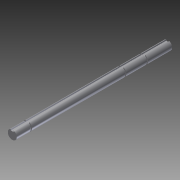
# Autodesk Inventor part: vertical drive shaft
Saved by Autodesk Inventor 2012 (Build 160160000, 160)
## iProperties
Created: 2012-07-07
Part Number: vertical drive shaft
Material: Default
Document SubType Name: Modeling
Designer: Bryce
Density: 1 g/cm^3
Author: Bryce
Autodesk Inventor part; units mm, degrees
sketch "Sketch1" plane through (0, 0, 0) normal (0, 0, 1) x (1, 0, 0)
  circle A0 centre (0, 0) radius 4.7625
  line L0 (-1.5875, 6.35) -> (1.5875, 6.35)
  line L1 (1.5875, 6.35) -> (1.5875, 3.175)
  line L2 (1.5875, 3.175) -> (-1.5875, 3.175)
  line L3 (-1.5875, 3.175) -> (-1.5875, 6.35)
  dimension "d0" = 9.525
  dimension "d43" = 3.175
  dimension "d44" = 3.175
  dimension "d45" = 1.5875
  dimension "d46" = 6.35
  constraints: 8 end point, 2 parallel, 1 centre point, 1 coincident, 1 horizontal, 1 perpendicular
  measures "d0" diameter of A0
  measures "d43" distance of L0.start L0.end
  measures "d44" distance of L0.end L1.end
  measures "d45" distance from line of point (0, 0) L1
  measures "d46" distance from line of point (0, 0) L0
extrude "Extrusion1" add sketch "Sketch1" along normal blind 165.05 contours A0 L3 L2 L1 | L1 L2 L3 A0
ref_plane "Work Plane6" through (0, 0, 176.4284) normal (0, 0, 1) x (1, 0, 0)
ref_plane "Work Plane12" through (0, 0, 148.9464) normal (0, 0, 1) x (1, 0, 0)
sketch "Sketch10" plane through (0, 0, 148.9464) normal (0, 0, 1) x (1, 0, 0)
  circle A0 centre (0, 0) radius 3.8481 projected
  circle A1 centre (0, 0) radius 4.7625 projected
extrude "Extrusion11" cut sketch "Sketch10" along normal blind 1.143
ref_plane "Work Plane13" through (0, 0, 49.7586) normal (0, 0, -1) x (-1, 0, 0)
sketch "Sketch11" plane through (0, 0, 49.7586) normal (0, 0, -1) x (-1, 0, 0)
  circle A0 centre (0, 0) radius 4.7625 projected
  circle A1 centre (0, 0) radius 3.8481 projected
  circle A2 centre (0, 0) radius 4.7625 projected
extrude "Extrusion12" cut sketch "Sketch11" along normal blind 1.143
ref_plane "Work Plane14" through (0, 0, 26.797) normal (0, 0, -1) x (-1, 0, 0)
sketch "Sketch12" plane through (0, 0, 26.797) normal (0, 0, -1) x (-1, 0, 0)
  circle A0 centre (0, 0) radius 3.8481 projected
  circle A1 centre (0, 0) radius 4.7625 projected
extrude "Extrusion13" cut sketch "Sketch12" along normal blind 1.143
ref_plane "Work Plane15" through (0, 0, 148.921) normal (0, 0, 1) x (1, 0, 0)
extrude "Extrusion14" cut sketch "Sketch1" along normal through all contours L1 L2 L3 A0 | A0 L3 L0 L1 picked at (-0.1794, 3.694)
equation "\"d44\" = d43"
equation "\"d45\" = 0.5 * d43"
equation "\"d46\" = 0.5 * d0 + 0.5 * d43"
body "Solid1"
